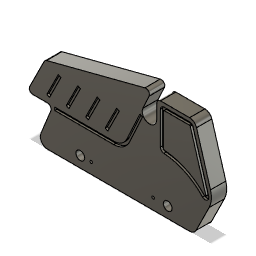
SchubLaster (Autodesk Fusion 360 design; units mm, degrees)
Autodesk Fusion 360 part; units mm, degrees
sketch "Skizze1" plane through (0, 0, 0) normal (0, 0, 1) x (1, 0, 0)
  circle A0 centre (0, 0) radius 4
  circle A1 centre (0, 0) radius 47.5
  circle A2 centre (0, 0) radius 6
  circle A3 centre (0, 0) radius 45
  line L0 (4.2426, 4.2426) -> (31.8198, 31.8198) construction
  line L1 (3.4762, 4.8904) -> (31.1048, 32.5191)
  line L2 (4.8904, 3.4762) -> (32.5191, 31.1048)
  line L3 (0, 6) -> (0, 45) construction
  line L4 (-1, 5.4889) -> (-1, 44.9889)
  line L5 (1, 7.0933) -> (1, 44.9889)
  line L6 (0, 45) -> (21.7929, 23.2071) construction
  line L7 (31.8198, 31.8198) -> (1, 31.8198) construction
  line L8 (1.2695, 44.9821) -> (22.4187, 23.8329)
  line L9 (-1, 44.9889) -> (21.2873, 22.7016)
  line L10 (32.5191, 31.1048) -> (1, 31.1048)
  line L11 (30.9094, 32.7048) -> (1, 32.7048)
  line L12 (13.1802, 31.8198) -> (2.2961, 5.5433) construction
  line L13 (1, 26.0411) -> (17.7067, 19.1209)
  line L14 (1, 23.8763) -> (16.176, 17.5902)
  line L15 (1, 7.0933) -> (1, 5.9161)
  line L16 (-1, 5.4889) -> (-1, 5.9161)
  line L17 (-19.5335, 40.5394) -> (-29.2734, 10.563)
  line L18 (-42.7975, 13.9058) -> (-15.3369, 27.8977) construction
  line L19 (-24.4575, 8.9982) -> (-12.7134, 22.7488)
  line L20 (-26.1895, 22.368) -> (-4.5624, 3.8967) construction
  line L21 (-2.7239, 5.346) -> (-20.4296, 40.0953) construction
  line L22 (-1.7948, 5.7253) -> (-19.5335, 40.5394)
  line L23 (-22.3987, 8.3292) -> (-11.7306, 20.8199)
  line L24 (-21.5526, 39.503) -> (-30.7951, 11.0574)
  line L25 (-6.4371, 3.143) -> (-5.3175, 2.7792)
  line L26 (-3.5769, 4.8173) -> (-21.3155, 39.6314)
  line L27 (-42.3882, 15.1076) -> (-15.7387, 28.6862)
  line L28 (-20.4296, 40.0953) -> (-29.9534, 10.7839) construction
  line L29 (-6.4371, 3.143) -> (-42.478, 14.8534)
  line L30 (-5.7063, 1.8541) -> (-42.7975, 13.9058) construction
  line L31 (-5.5293, 0.7451) -> (-43.096, 12.9513)
  line L32 (-43.096, 12.9513) -> (-15.0123, 27.2606)
  line L33 (-5.5293, 0.7451) -> (-5.9355, 0.8771)
  line L34 (-44.5914, -6.0501) -> (-19.092, -24.5766)
  line L35 (-26.4503, -36.4058) -> (-31.2716, -5.9654) construction
  line L36 (-16.1156, -20.4799) -> (-25.564, -5.0614)
  line L37 (-29.3662, -17.9956) -> (-5.1158, -3.135) construction
  line L38 (-5.9261, -0.9386) -> (-44.446, -7.0396) construction
  line L39 (-5.9997, 0.0622) -> (-44.5914, -6.0501)
  line L40 (-14.8432, -18.7285) -> (-23.4259, -4.7228)
  line L41 (-44.2297, -8.2907) -> (-20.0324, -25.871)
  line L42 (-4.9783, -5.1508) -> (-4.2864, -4.1984)
  line L43 (-5.6868, -1.9132) -> (-44.2786, -8.0255)
  line L44 (-27.4669, -35.6451) -> (-32.1458, -6.1039)
  line L45 (-44.446, -7.0396) -> (-19.5122, -25.155) construction
  line L46 (-4.9783, -5.1508) -> (-27.2528, -35.809)
  line L47 (-3.5267, -4.8541) -> (-26.4503, -36.4058) construction
  line L48 (-2.4173, -5.0284) -> (-25.6348, -36.9846)
  line L49 (-25.6348, -36.9846) -> (-30.5655, -5.8536)
  line L50 (-2.4173, -5.0284) -> (-2.6684, -5.374)
  line L51 (-8.0255, -44.2786) -> (17.4739, -25.7521)
  line L52 (26.4503, -36.4058) -> (-3.99, -31.5845) construction
  line L53 (14.4975, -21.6555) -> (-3.086, -25.8769)
  line L54 (8.0402, -33.4899) -> (1.4007, -5.8342) construction
  line L55 (-0.9386, -5.9261) -> (-7.0396, -44.446) construction
  line L56 (-1.9132, -5.6868) -> (-8.0255, -44.2786)
  line L57 (13.2251, -19.9041) -> (-2.7474, -23.7388)
  line L58 (-5.7828, -44.6269) -> (18.4144, -27.0466)
  line L59 (3.3603, -6.3264) -> (2.6684, -5.374)
  line L60 (0.0622, -5.9997) -> (-6.0501, -44.5914)
  line L61 (25.4127, -37.1375) -> (-4.1285, -32.4586)
  line L62 (-7.0396, -44.446) -> (17.8942, -26.3305) construction
  line L63 (3.3603, -6.3264) -> (25.6348, -36.9846)
  line L64 (3.5267, -4.8541) -> (26.4503, -36.4058) construction
  line L65 (4.0353, -3.8528) -> (27.2528, -35.809)
  line L66 (27.2528, -35.809) -> (-3.8782, -30.8783)
  line L67 (4.0353, -3.8528) -> (4.2864, -4.1984)
  line L68 (39.6314, -21.3155) -> (29.8915, 8.6609)
  line L69 (42.7975, 13.9058) -> (28.8056, -13.5549) construction
  line L70 (25.0756, 7.0961) -> (23.6568, -10.9314)
  line L71 (34.3353, -2.7022) -> (5.9815, -0.4708) construction
  line L72 (5.346, -2.7239) -> (40.0953, -20.4296) construction
  line L73 (4.8173, -3.5769) -> (39.6314, -21.3155)
  line L74 (23.0167, 6.4271) -> (21.7279, -9.9486)
  line L75 (40.6557, -19.2903) -> (31.4132, 9.1553)
  line L76 (7.0551, 1.2409) -> (5.9355, 0.8771)
  line L77 (5.7253, -1.7948) -> (40.5394, -19.5335)
  line L78 (43.1728, 12.6928) -> (29.5942, -13.9567)
  line L79 (40.0953, -20.4296) -> (30.5715, 8.8818) construction
  line L80 (7.0551, 1.2409) -> (43.096, 12.9513)
  line L81 (5.7063, 1.8541) -> (42.7975, 13.9058) construction
  line L82 (4.9112, 2.6472) -> (42.478, 14.8534)
  line L83 (42.478, 14.8534) -> (28.1686, -13.2303)
  line L84 (4.9112, 2.6472) -> (5.3175, 2.7792)
  dimension "d1" = 8
  dimension "d2" = 95
  dimension "d3" = 12
  dimension "d4" = 2.5
  dimension "d6" = 2
  dimension "d7" = 2
  dimension "d9" = 45
  dimension "d10" = 1.6
  dimension "d11" = 1.6
  dimension "d12" = 2
  dimension "d13" = 10
  dimension "d15" = 360
  constraint coincident A0.centre A1.centre
  constraint concentric A0 A3
  constraint coincident A2 L0.start
  constraint coincident A3 L0.end
  constraint coincident A0.centre L0
  constraint coincident A2 L1.start
  constraint coincident A3 L1.end
  constraint coincident A2 L2.start
  constraint coincident A3 L2.end
  constraint parallel L0 L2
  constraint parallel L0 L1
  constraint symmetric L0 L1 L2
  constraint coincident A2 L3.start
  constraint coincident A3 L3.end
  constraint vertical L3
  constraint coincident A0.centre L3
  constraint coincident A3 L4.end
  constraint parallel L3 L4
  constraint coincident A3 L5.end
  constraint parallel L3 L5
  constraint coincident L1 L6.end
  constraint perpendicular L1 L6
  constraint coincident L5 L7.end
  constraint perpendicular L5 L7
  constraint coincident L1 L8.end
  constraint perpendicular L1 L8
  constraint coincident L1 L9.end
  constraint perpendicular L1 L9
  constraint coincident L5 L10.end
  constraint perpendicular L5 L10
  constraint coincident A3 L11.start
  constraint coincident L5 L11.end
  constraint perpendicular L5 L11
  constraint coincident L4.end L9
  constraint coincident L6 L12.start
  constraint coincident L7 L12.start
  constraint coincident A2 L12.end
  constraint coincident A0.centre L12
  constraint midpoint L5 L13.start
  constraint coincident L1 L13.end
  constraint coincident L5 L14.start
  constraint coincident L1 L14.end
  constraint parallel L13 L14
  constraint perpendicular L12 L13
  constraint coincident A2 L15.end
  constraint parallel L5 L15
  constraint coincident A2 L16.end
  constraint parallel L4 L16
  constraint coincident A3 L8.start
  measures "d1" diameter of A0
  measures "d2" diameter of A1
  measures "d3" diameter of A2
  measures "d4" distance of A1 A3
  measures "d6" distance of L1 L2
  measures "d7" distance of L4 L5
  measures "d9" angle of L1 L5
  measures "d10" distance of L10 L11
  measures "d11" distance of L8 L9
  measures "d12" distance of L13 L14
  measures "d13" distance of L12.start L13
extrude "Extrusion1" add sketch "Skizze1" along normal blind 20 contours A1 | A2 | A2 L76 L80 L82 L83 | A2 L68 L73 L77 | L70 L74 L77 L80 | A2 L1 L2 L10 | A3 L80 L83 | A2 L59 L63 L65 L66 | A3 L68 L77 | A3 L1 L10 | A3 L75 L78 L80 L83 | A3 L63 L66 | A3 L68 L75 L77 L78 | L68 L77 L78 L83 | A2 L4 L5 L9 L15 | L1 L5 L13 L14 | A3 L1 L8 L10 L11 | L68 L75 L80 L83 | L68 L75 L78 L83 | A2 L51 L56 L60 | A3 L58 L61 L63 L66 | L1 L8 L9 L10 | L8 L9 L10 L11 | L53 L57 L60 L63 | L51 L58 L63 L66 | L51 L58 L61 L66 | A2 L17 L22 L26 | A3 L5 L9 | A3 L5 L8 L9 L11 | L5 L9 L10 L11 | A2 L42 L46 L48 L49 | A3 L51 L60 | A3 L51 L58 L60 L61 | L51 L60 L61 L66 | A3 L17 L26 | A3 L46 L49 | A2 L25 L29 L31 L32 | L19 L23 L26 L29 | A3 L17 L24 L26 L27 | A2 L34 L39 L43 | A3 L41 L44 L46 L49 | L17 L26 L27 L32 | L17 L24 L27 L32 | L36 L40 L43 L46 | L34 L41 L46 L49 | L34 L41 L44 L49 | A3 L29 L32 | A3 L24 L27 L29 L32 | L17 L24 L29 L32 | A3 L34 L43 | A3 L34 L41 L43 L44 | L34 L43 L44 L49 makes body 1
copy_body "Körper->Berechn1" bodies 1 removing the originals makes body 2 in component "Component"
sketch "Skizze2" plane through (0, 0, 0) normal (0, 1, 0) x (1, 0, 0)
  circle A0 centre (250, 0) radius 42.5
  dimension "d27" = 85
  measures "d27" diameter of A0
sketch "Skizze1 (2)" plane through (0, 0, 0) normal (0, 0, 1) x (1, 0, 0) in component "Component'"
  circle A0 centre (0, 0) radius 6
  circle A1 centre (-120, 0) radius 6
  line L0 (-165, -15) -> (30, -15)
  arc A2 (30, -15) -> (38.9581, -9.4444) centre (30, -5) ccw
  line L1 (38.9581, -9.4444) -> (56.8742, 26.6667)
  arc A3 (56.8742, 26.6667) -> (58.7494, 48.5714) centre (30, 40) ccw
  line L2 (58.7494, 48.5714) -> (39.5831, 112.8571)
  arc A4 (39.5831, 112.8571) -> (30, 120) centre (30, 110) ccw
  line L3 (30, 120) -> (-10, 120)
  arc A5 (-10, 120) -> (-15, 115) centre (-10, 115) ccw
  line L4 (-15, 115) -> (-15, 95)
  arc A6 (-34.0829, 99.1834) -> (-15, 95) centre (-25, 95) ccw
  line L5 (-34.0829, 99.1834) -> (-25.4586, 117.9083)
  arc A7 (-25.4586, 117.9083) -> (-31.2548, 124.84) centre (-30, 120) ccw
  line L6 (-31.2548, 124.84) -> (-166.2548, 89.84)
  arc A8 (-166.2548, 89.84) -> (-169.4721, 87.2361) centre (-165, 85) ccw
  line L7 (-169.4721, 87.2361) -> (-189.4721, 47.2361)
  arc A9 (-189.4721, 47.2361) -> (-185, 40) centre (-185, 45) ccw
  line L8 (-185, 40) -> (-165, 40)
  arc A10 (-160.3649, 33.125) -> (-165, 40) centre (-165, 35) ccw
  line L9 (-160.3649, 33.125) -> (-174.2702, -1.25)
  arc A11 (-174.2702, -1.25) -> (-165, -15) centre (-165, -5) ccw
  dimension "d133" = 12
  dimension "d134" = 120
  dimension "d135" = 15
  dimension "d136" = 45
  dimension "d137" = 30
  dimension "d138" = 30
  dimension "d139" = 40
  dimension "d140" = 10
  dimension "d141" = 5
  dimension "d142" = 30
  dimension "d143" = 80
  dimension "d144" = 20
  dimension "d145" = 10
  dimension "d146" = 25
  dimension "d147" = 20
  dimension "d148" = 40
  dimension "d149" = 20
  dimension "d150" = 40
  constraint coincident A0.centre origin
  constraint equal A0 A1
  constraint horizontal A0.centre A1.centre
  constraint horizontal L0
  constraint tangent L0 A2
  constraint tangent L1 A3
  constraint tangent A3 L2
  constraint tangent L2 A4
  constraint horizontal L3
  constraint tangent L3 A5
  constraint perpendicular L3 L4
  constraint tangent L4 A6
  constraint tangent L5 A7
  constraint tangent L6 A8
  constraint tangent A8 L7
  constraint tangent L7 A9
  constraint horizontal L8
  constraint tangent L8 A10
  constraint tangent L9 A11
  constraint tangent A4 L3
  constraint tangent A2 L1
  constraint tangent L0 A11
  constraint tangent A10 L9
  constraint tangent A9 L8
  constraint tangent A7 L6
  constraint tangent A6 L5
  constraint tangent A5 L4
  constraint equal A2 A11
  constraint equal A9 A10
  constraint equal A8 A10
  constraint equal A7 A10
  constraint equal A2 A6
  constraint equal A5 A10
  constraint equal A2 A4
  constraint vertical A2.centre A4.centre
  constraint vertical A10.centre A11.centre
  constraint vertical A8.centre A10.centre
  measures "d133" diameter of A0
  measures "d134" distance of A0.centre A1.centre
  measures "d135" distance of A0.centre L0
  measures "d136" horizontal distance of A1.centre A11.centre
  measures "d137" horizontal distance of A0.centre A2.centre
  measures "d138" radius of A3
  measures "d139" vertical distance of A0.centre A3.centre
  measures "d140" radius of A2
  measures "d141" radius of A10
  measures "d142" horizontal distance of A0.centre A3.centre
  measures "d143" distance of A3.centre L3
  measures "d144" distance of A5.end L4.end
  measures "d145" horizontal distance of A0.centre A5.centre
  measures "d146" vertical distance of A6.centre A7.centre
  measures "d147" horizontal distance of A5.centre A7.centre
  measures "d148" distance of A10.centre A11.centre
  measures "d149" horizontal distance of A9.centre A10.centre
  measures "d150" vertical distance of A8.centre A9.centre
extrude "Extrusion1'" add sketch "Skizze1 (2)" along normal blind 21 separate body makes body 3 in component "Component'"
sketch "Skizze2 (2)" plane through (0, 0, 0) normal (0, 0, -1) x (-1, 0, 0) in component "Component'"
  circle A0 centre (0, 0) radius 6
  circle A1 centre (120, 0) radius 6
  line L0 (174.2702, -1.25) -> (160.3649, 33.125)
  arc A2 (165, 40) -> (160.3649, 33.125) centre (165, 35) ccw
  line L1 (165, 40) -> (185, 40)
  arc A3 (185, 40) -> (189.4721, 47.2361) centre (185, 45) ccw
  line L2 (189.4721, 47.2361) -> (169.4721, 87.2361)
  arc A4 (169.4721, 87.2361) -> (166.2548, 89.84) centre (165, 85) ccw
  line L3 (166.2548, 89.84) -> (31.2548, 124.84)
  arc A5 (31.2548, 124.84) -> (25.4586, 117.9083) centre (30, 120) ccw
  line L4 (25.4586, 117.9083) -> (34.0829, 99.1834)
  arc A6 (15, 95) -> (34.0829, 99.1834) centre (25, 95) ccw
  line L5 (15, 95) -> (15, 115)
  arc A7 (15, 115) -> (10, 120) centre (10, 115) ccw
  line L6 (10, 120) -> (-30, 120)
  arc A8 (-30, 120) -> (-39.5831, 112.8571) centre (-30, 110) ccw
  line L7 (-39.5831, 112.8571) -> (-58.7494, 48.5714)
  arc A9 (-58.7494, 48.5714) -> (-56.8742, 26.6667) centre (-30, 40) ccw
  line L8 (-56.8742, 26.6667) -> (-38.9581, -9.4444)
  arc A10 (-38.9581, -9.4444) -> (-30, -15) centre (-30, -5) ccw
  line L9 (-30, -15) -> (165, -15)
  arc A11 (165, -15) -> (174.2702, -1.25) centre (165, -5) ccw
  line L10 (185, 40) -> (74.1495, 40)
  arc A12 (55.9837, 51.6332) -> (74.1495, 40) centre (74.1495, 60) ccw
  line L11 (55.9837, 51.6332) -> (34.0829, 99.1834)
  line L12 (185, 36) -> (74.1495, 36)
  arc A13 (52.3505, 49.9598) -> (74.1495, 36) centre (74.1495, 60) ccw
  line L13 (52.3506, 49.9598) -> (30.4497, 97.5101)
  line L14 (150.1826, 81.0938) -> (165.8351, 49.7889)
  line L15 (165.8351, 49.7889) -> (162.2574, 48)
  line L16 (162.2574, 48) -> (146.6049, 79.305)
  line L17 (146.6049, 79.305) -> (150.1826, 81.0938)
  line L18 (135.5907, 48) -> (119.9382, 79.305)
  line L19 (119.9382, 79.305) -> (123.5159, 81.0938)
  line L20 (139.1684, 49.7889) -> (135.5907, 48)
  line L21 (123.5159, 81.0938) -> (139.1684, 49.7889)
  line L22 (108.924, 48) -> (93.2715, 79.305)
  line L23 (93.2715, 79.305) -> (96.8493, 81.0938)
  line L24 (112.5017, 49.7889) -> (108.924, 48)
  line L25 (96.8493, 81.0938) -> (112.5017, 49.7889)
  line L26 (82.2574, 48) -> (66.6049, 79.305)
  line L27 (66.6049, 79.305) -> (70.1826, 81.0938)
  line L28 (85.8351, 49.7889) -> (82.2574, 48)
  line L29 (70.1826, 81.0938) -> (85.8351, 49.7889)
  line L30 (5, 115) -> (-30, 115)
  arc A14 (-30, 115) -> (-34.7916, 111.4286) centre (-30, 110) ccw
  line L31 (-34.7916, 111.4286) -> (-56.2082, 39.5951)
  arc A15 (-56.2082, 39.5951) -> (-55.8956, 35.9443) centre (-51.4166, 38.1665) ccw
  line L32 (-55.8956, 35.9443) -> (-55.8702, 35.893)
  arc A16 (-55.8702, 35.893) -> (-47.7314, 34.7084) centre (-51.3911, 38.1152) ccw
  arc A17 (5.3426, 60.0118) -> (-47.7314, 34.7084) centre (10.8246, -19.8002) ccw
  arc A18 (5.3426, 60.0118) -> (10, 65) centre (5, 65) ccw
  line L33 (10, 65) -> (10, 110)
  arc A19 (10, 110) -> (5, 115) centre (5, 110) ccw
  line L34 (34.6332, 88.4272) -> (38.2663, 90.1005)
  line L35 (155, 36) -> (155, 40)
  line L36 (5, 111) -> (-30, 111)
  arc A20 (-30, 111) -> (-30.9583, 110.2857) centre (-30, 110) ccw
  line L37 (-30.9583, 110.2857) -> (-52.3749, 38.4523)
  arc A21 (-52.3749, 38.4523) -> (-52.3124, 37.7221) centre (-51.4166, 38.1665) ccw
  line L38 (-52.3124, 37.7221) -> (-52.287, 37.6708)
  arc A22 (-52.287, 37.6708) -> (-50.6592, 37.4339) centre (-51.3911, 38.1152) ccw
  arc A23 (5.0685, 64.0024) -> (-50.6592, 37.4339) centre (10.8246, -19.8002) ccw
  arc A24 (5.0685, 64.0024) -> (6, 65) centre (5, 65) ccw
  line L39 (6, 65) -> (6, 110)
  arc A25 (6, 110) -> (5, 111) centre (5, 110) ccw
  dimension "d153" = 20
  dimension "d154" = -4
  dimension "d155" = 20
  dimension "d156" = 4
  dimension "d157" = 8
  dimension "d158" = 35
  dimension "d161" = -80
  dimension "d162" = 0
  dimension "d164" = 5
  dimension "d165" = 5
  dimension "d166" = 5
  dimension "d167" = 5
  dimension "d168" = 5
  dimension "d171" = 45
  dimension "d172" = 75
  dimension "d173" = -4
  dimension "d174" = 10
  dimension "d175" = 30
  dimension "d181" = 5
  dimension "d182" = 80
  constraint coincident L1.end A3.start
  constraint tangent L10 A12
  constraint coincident L4.end A6.end
  constraint tangent A12 L11
  constraint collinear L4 L11
  constraint collinear L1 L10
  constraint perpendicular L14 L15
  constraint perpendicular L15 L16
  constraint parallel L2 L14
  constraint perpendicular L14 L17
  constraint perpendicular L5 L30
  constraint tangent L30 A14
  constraint tangent L31 A15
  constraint tangent L32 A16
  constraint tangent A16 A17
  constraint tangent A17 A18
  constraint vertical L33
  constraint tangent L33 A19
  constraint tangent A14 L31
  constraint tangent A15 L32
  constraint tangent A18 L33
  constraint tangent L30 A19
  constraint parallel L7 L31
  constraint parallel L8 L32
  constraint equal A14 A16
  constraint equal A16 A18
  constraint equal A14 A19
  constraint coincident L13 L34.start
  constraint coincident L11 L34.end
  constraint perpendicular L11 L34
  constraint coincident L12 L35.start
  constraint coincident L10 L35.end
  constraint perpendicular L10 L35
  measures "d153" radius of A12
  measures "d155" distance of L2 L14
  measures "d156" distance of L14.end L15.end
  measures "d157" distance of L10 L15.end
  measures "d158" distance of L14.start L14.end
  measures "d164" radius of A14
  measures "d165" distance of L5 L33
  measures "d166" distance of L7 L31
  measures "d167" distance of L8 L32
  measures "d168" radius of A15
  measures "d171" distance of A18.centre A19.centre
  measures "d172" distance of A8.centre A16.centre
  measures "d174" distance of L4.end L34
  measures "d175" distance of L12.start L35.start
  measures "d181" distance of L6 L30
  measures "d182" radius of A17
extrude "Extrusion2" cut sketch "Skizze2 (2)" against normal blind 3 contours L10 A12 L11 L12 A13 L13 L34 L35 | L14 L15 L16 L17 | L18 L19 L20 L21 | L22 L23 L24 L25 | L26 L27 L28 L29 | L30 A14 L31 A15 L32 A16 A17 A18 L33 A19 bodies 3 in component "Component'"
sketch "Skizze3" plane through (0, 0, 21) normal (0, 0, 1) x (1, 0, 0) in component "Component'"
  circle A0 centre (0, 0) radius 6
  circle A1 centre (-120, 0) radius 6
  line L0 (-160.3649, 33.125) -> (-174.2702, -1.25)
  arc A2 (-174.2702, -1.25) -> (-165, -15) centre (-165, -5) ccw
  line L1 (-165, -15) -> (30, -15)
  arc A3 (30, -15) -> (38.9581, -9.4444) centre (30, -5) ccw
  line L2 (38.9581, -9.4444) -> (56.8742, 26.6667)
  arc A4 (56.8742, 26.6667) -> (58.7494, 48.5714) centre (30, 40) ccw
  line L3 (58.7494, 48.5714) -> (39.5831, 112.8571)
  arc A5 (39.5831, 112.8571) -> (30, 120) centre (30, 110) ccw
  line L4 (30, 120) -> (-10, 120)
  arc A6 (-10, 120) -> (-15, 115) centre (-10, 115) ccw
  line L5 (-15, 115) -> (-15, 95)
  arc A7 (-34.0829, 99.1834) -> (-15, 95) centre (-25, 95) ccw
  line L6 (-34.0829, 99.1834) -> (-25.4586, 117.9083)
  arc A8 (-25.4586, 117.9083) -> (-31.2548, 124.84) centre (-30, 120) ccw
  line L7 (-31.2548, 124.84) -> (-166.2548, 89.84)
  arc A9 (-166.2548, 89.84) -> (-169.4721, 87.2361) centre (-165, 85) ccw
  line L8 (-169.4721, 87.2361) -> (-189.4721, 47.2361)
  arc A10 (-189.4721, 47.2361) -> (-185, 40) centre (-185, 45) ccw
  line L9 (-185, 40) -> (-165, 40)
  arc A11 (-160.3649, 33.125) -> (-165, 40) centre (-165, 35) ccw
  arc A12 (-6, 65) -> (-5.0685, 64.0024) centre (-5, 65) ccw
  arc A13 (50.6592, 37.4339) -> (-5.0685, 64.0024) centre (-10.8246, -19.8002) ccw
  arc A14 (50.6592, 37.4339) -> (52.287, 37.6708) centre (51.3911, 38.1152) ccw
  line L10 (52.287, 37.6708) -> (52.3124, 37.7221)
  arc A15 (52.3124, 37.7221) -> (52.3749, 38.4523) centre (51.4166, 38.1665) ccw
  line L11 (52.3749, 38.4523) -> (30.9583, 110.2857)
  arc A16 (30.9583, 110.2857) -> (30, 111) centre (30, 110) ccw
  line L12 (30, 111) -> (-5, 111)
  arc A17 (-5, 111) -> (-6, 110) centre (-5, 110) ccw
  line L13 (-6, 110) -> (-6, 65)
  arc A18 (-10, 65) -> (-5.3426, 60.0118) centre (-5, 65) ccw
  line L14 (-10, 65) -> (-10, 110)
  arc A19 (-5, 115) -> (-10, 110) centre (-5, 110) ccw
  line L15 (-5, 115) -> (30, 115)
  arc A20 (34.7916, 111.4286) -> (30, 115) centre (30, 110) ccw
  line L16 (34.7916, 111.4286) -> (56.2082, 39.5951)
  arc A21 (55.8956, 35.9443) -> (56.2082, 39.5951) centre (51.4166, 38.1665) ccw
  line L17 (55.8956, 35.9443) -> (55.8702, 35.893)
  arc A22 (47.7314, 34.7084) -> (55.8702, 35.893) centre (51.3911, 38.1152) ccw
  arc A23 (47.7314, 34.7084) -> (-5.3426, 60.0118) centre (-10.8246, -19.8002) ccw
  arc A24 (-74.1495, 36) -> (-52.3505, 49.9598) centre (-74.1495, 60) ccw
  line L18 (-74.1495, 36) -> (-155, 36)
  line L19 (-155, 36) -> (-155, 40)
  line L20 (-155, 40) -> (-74.1495, 40)
  arc A25 (-74.1495, 40) -> (-55.9837, 51.6332) centre (-74.1495, 60) ccw
  line L21 (-55.9837, 51.6332) -> (-38.2663, 90.1005)
  line L22 (-38.2663, 90.1005) -> (-34.6332, 88.4272)
  line L23 (-34.6332, 88.4272) -> (-52.3506, 49.9598)
  line L24 (-70.1826, 81.0938) -> (-66.6049, 79.305)
  line L25 (-66.6049, 79.305) -> (-82.2574, 48)
  line L26 (-82.2574, 48) -> (-85.8351, 49.7889)
  line L27 (-85.8351, 49.7889) -> (-70.1826, 81.0938)
  line L28 (-96.8493, 81.0938) -> (-93.2715, 79.305)
  line L29 (-93.2715, 79.305) -> (-108.924, 48)
  line L30 (-108.924, 48) -> (-112.5017, 49.7889)
  line L31 (-112.5017, 49.7889) -> (-96.8493, 81.0938)
  line L32 (-123.5159, 81.0938) -> (-119.9382, 79.305)
  line L33 (-119.9382, 79.305) -> (-135.5907, 48)
  line L34 (-135.5907, 48) -> (-139.1684, 49.7889)
  line L35 (-139.1684, 49.7889) -> (-123.5159, 81.0938)
  line L36 (-146.6049, 79.305) -> (-162.2574, 48)
  line L37 (-162.2574, 48) -> (-165.8351, 49.7889)
  line L38 (-165.8351, 49.7889) -> (-150.1826, 81.0938)
  line L39 (-150.1826, 81.0938) -> (-146.6049, 79.305)
extrude "Extrusion3" cut sketch "Skizze3" against normal blind 3 contours A18 L14 A19 L15 A20 L16 A21 L17 A22 A23 | A24 L18 L19 L20 A25 L21 L22 L23 | L24 L25 L26 L27 | L28 L29 L30 L31 | L32 L33 L34 L35 | L36 L37 L38 L39 bodies 3 in component "Component'"
sketch "Skizze4" plane through (0, 0, 0) normal (0, 0, -1) x (-1, 0, 0) in component "Component'"
  line L0 (174.2702, -1.25) -> (160.3649, 33.125)
  arc A0 (165, 40) -> (160.3649, 33.125) centre (165, 35) ccw
  line L1 (165, 40) -> (185, 40)
  arc A1 (185, 40) -> (189.4721, 47.2361) centre (185, 45) ccw
  line L2 (189.4721, 47.2361) -> (169.4721, 87.2361)
  arc A2 (169.4721, 87.2361) -> (166.2548, 89.84) centre (165, 85) ccw
  line L3 (166.2548, 89.84) -> (31.2548, 124.84)
  arc A3 (31.2548, 124.84) -> (25.4586, 117.9083) centre (30, 120) ccw
  line L4 (25.4586, 117.9083) -> (34.0829, 99.1834)
  arc A4 (15, 95) -> (34.0829, 99.1834) centre (25, 95) ccw
  line L5 (15, 95) -> (15, 115)
  arc A5 (15, 115) -> (10, 120) centre (10, 115) ccw
  line L6 (10, 120) -> (-30, 120)
  arc A6 (-30, 120) -> (-39.5831, 112.8571) centre (-30, 110) ccw
  line L7 (-39.5831, 112.8571) -> (-58.7494, 48.5714)
  arc A7 (-58.7494, 48.5714) -> (-56.8742, 26.6667) centre (-30, 40) ccw
  line L8 (-56.8742, 26.6667) -> (-38.9581, -9.4444)
  arc A8 (-38.9581, -9.4444) -> (-30, -15) centre (-30, -5) ccw
  line L9 (-30, -15) -> (165, -15)
  arc A9 (165, -15) -> (174.2702, -1.25) centre (165, -5) ccw
  circle A10 centre (0, 0) radius 6
  circle A11 centre (120, 0) radius 6
  line L10 (165.8351, 49.7889) -> (162.2574, 48)
  line L11 (162.2574, 48) -> (146.6049, 79.305)
  line L12 (146.6049, 79.305) -> (150.1826, 81.0938)
  line L13 (150.1826, 81.0938) -> (165.8351, 49.7889)
  line L14 (155, 36) -> (74.1495, 36)
  arc A12 (52.3505, 49.9598) -> (74.1495, 36) centre (74.1495, 60) ccw
  line L15 (52.3505, 49.9598) -> (34.6332, 88.4272)
  line L16 (34.6332, 88.4272) -> (38.2663, 90.1005)
  line L17 (38.2663, 90.1005) -> (55.9837, 51.6332)
  arc A13 (55.9837, 51.6332) -> (74.1495, 40) centre (74.1495, 60) ccw
  line L18 (74.1495, 40) -> (155, 40)
  line L19 (155, 40) -> (155, 36)
  line L20 (82.2574, 48) -> (66.6049, 79.305)
  line L21 (66.6049, 79.305) -> (70.1826, 81.0938)
  line L22 (70.1826, 81.0938) -> (85.8351, 49.7889)
  line L23 (85.8351, 49.7889) -> (82.2574, 48)
  line L24 (135.5907, 48) -> (119.9382, 79.305)
  line L25 (119.9382, 79.305) -> (123.5159, 81.0938)
  line L26 (123.5159, 81.0938) -> (139.1684, 49.7889)
  line L27 (139.1684, 49.7889) -> (135.5907, 48)
  line L28 (10, 110) -> (10, 65)
  arc A14 (5.3426, 60.0118) -> (10, 65) centre (5, 65) ccw
  arc A15 (5.3426, 60.0118) -> (-47.7314, 34.7084) centre (10.8246, -19.8002) ccw
  arc A16 (-55.8702, 35.893) -> (-47.7314, 34.7084) centre (-51.3911, 38.1152) ccw
  line L29 (-55.8702, 35.893) -> (-55.8956, 35.9443)
  arc A17 (-56.2082, 39.5951) -> (-55.8956, 35.9443) centre (-51.4166, 38.1665) ccw
  line L30 (-56.2082, 39.5951) -> (-34.7916, 111.4286)
  arc A18 (-30, 115) -> (-34.7916, 111.4286) centre (-30, 110) ccw
  line L31 (-30, 115) -> (5, 115)
  arc A19 (10, 110) -> (5, 115) centre (5, 110) ccw
  line L32 (108.924, 48) -> (93.2715, 79.305)
  line L33 (93.2715, 79.305) -> (96.8493, 81.0938)
  line L34 (96.8493, 81.0938) -> (112.5017, 49.7889)
  line L35 (112.5017, 49.7889) -> (108.924, 48)
  circle A20 centre (20, 0) radius 1.75
  circle A21 centre (105, 0) radius 1.75
  dimension "d191" = 3.5
  dimension "d192" = 3.5
  dimension "d193" = 20
  dimension "d194" = 85
  constraint horizontal A10.centre A20.centre
  constraint horizontal A20.centre A21.centre
  measures "d191" diameter of A20
  measures "d192" diameter of A21
  measures "d193" distance of A10.centre A20.centre
  measures "d194" distance of A20.centre A21.centre
extrude "Extrusion4" cut sketch "Skizze4" against normal blind 30 contours A20 | A21 bodies 3 in component "Component'"
component "Component" placed x (1, 0, 0) y (0, 1, 0) z (0, 0, 1) at (0, 0, 10)
component "Component" placed x (1, 0, 0) y (0, 1, 0) z (0, 0, 1) at (-120, 0, 10)
component "Component" placed x (1, 0, 0) y (0, 1, 0) z (0, 0, 1) at (0, 0, -50)
component "Component" placed x (1, 0, 0) y (0, 1, 0) z (0, 0, 1) at (-120, 0, -50)
component "Component'" placed x (1, 0, 0) y (0, 1, 0) z (0, 0, 1) at (0, 0, -20)
equation "d6 = d7"
equation "d11 = d10"
equation "d142 = d137"
equation "d150 = d148"
equation "d163 = 5.00 mm"
equation "d165 = d163"
equation "d166 = d163"
equation "d167 = d163"
